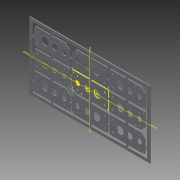
# Autodesk Inventor part: Granny Gearbox Input Plate Routing Template (9-up)
Saved by Autodesk Inventor 2015 (Build 190159000, 159)
## iProperties
Created: 2016-02-25
Part Number: Granny Gearbox Input Plate Routing Template (9-up)
Material: Generic
Document SubType Name: Modeling
Designer: sethbattis
Density: 1 g/cm^3
Appearance: Default
Author: sethbattis
Autodesk Inventor part; units mm, degrees
ref_plane "YZ Plane" through (0, 0, 0) normal (1, 0, 0) x (0, 1, 0)
ref_plane "XZ Plane" through (0, 0, 0) normal (0, 1, 0) x (-1, 0, 0)
ref_plane "XY Plane" through (0, 0, 0) normal (0, 0, 1) x (1, 0, 0)
derived "Granny Gearbox Input Plate.ipt"
feature "Solid1::Granny Gearbox Input Plate.ipt" [suppressed]
sketch "Shaft Alignment" plane through (0, 0, 0) normal (0, 0, 1) x (1, 0, 0)
  line L0 (-40.7035, -5.5985) -> (-0.0001, -11.1125) construction
  line L1 (-35.1409, -0.031) -> (-35.1353, -6.3528) construction
  line L2 (-11.1125, -0.0098) -> (-11.104, -9.6083) construction
  line L3 (0, 11.1125) -> (43.74, 13.9583) construction
  line L4 (-40.7035, -5.5985) -> (-46.2661, -5.5985) construction
  line L5 (-40.7035, -19.8733) -> (-46.2661, -19.8733) construction
  line L6 (-40.7035, 19.8015) -> (-46.2661, 19.8015) construction
  line L7 (-40.7035, 5.5267) -> (-46.2661, 5.5267) construction
  line L8 (-46.2661, 25.3641) -> (-46.2661, -25.4359) construction
  line L9 (-40.7035, 25.3641) -> (-40.7035, -25.4359) construction
  line L10 (-40.7035, -0.0359) -> (0, 0) construction
  line L11 (0, 0) -> (40.6908, 0) construction
  line L12 (11.1125, 0) -> (11.1125, 11.8355) construction
  line L13 (26.4033, 0) -> (26.4033, 12.8304) construction
  circle A0 centre (-40.7035, 25.3641) radius 5.5626
  circle A1 centre (-40.7035, -25.4359) radius 5.5626
  circle A2 centre (40.6908, 0) radius 14.2875
  circle A3 centre (0, 0) radius 11.1125
  circle A4 centre (-40.7035, -0.0359) radius 5.5626
  point P0 (-33.5787, -27.5177)
sketch "New Mounting Holes" plane through (0, 0, 0) normal (0, 0, 1) x (1, 0, 0)
  circle A0 centre (-40.7035, -0.0359) radius 31.75 construction
  circle A1 centre (40.6908, 0) radius 36.195 construction
  circle A2 centre (0, 0) radius 36.195 construction
  line L0 (-57.7242, 30.4609) -> (-55.8383, 30.4609) construction
  line L1 (-57.7242, 30.4609) -> (-57.7242, 28.575) construction
  circle A3 centre (-57.7242, 30.4609) radius 3.175
  circle A4 centre (-24.3812, -30.912) radius 3.175
  line L2 (-65.3633, -38.1) -> (-65.3633, 38.1) construction
  line L3 (87.0367, -38.1) -> (-65.3633, -38.1) construction
  line L4 (87.0367, 38.1) -> (87.0367, -38.1) construction
  line L5 (-65.3633, 38.1) -> (87.0367, 38.1) construction
  line L6 (-55.8383, 38.1) -> (-55.8383, -38.1) construction
  line L7 (-65.3633, 28.575) -> (87.0367, 28.575) construction
  line L8 (-65.3633, -28.575) -> (87.0367, -28.575) construction
  line L9 (77.5117, 38.1) -> (77.5117, -38.1) construction
  circle A5 centre (74.3367, 23.3553) radius 3.175
  circle A6 centre (74.3367, -23.3553) radius 3.175
sketch "Labels" plane through (0, 0, 0) normal (0, 0, 1) x (1, 0, 0)
  circle A0 centre (-40.7035, -0.0359) radius 5.5626
  circle A1 centre (-40.7035, 25.3641) radius 5.5626
  circle A2 centre (-40.7035, -25.4359) radius 5.5626
  circle A3 centre (0, 0) radius 11.1125
  circle A4 centre (40.6908, 0) radius 14.2875
  line L0 (-5.8677, 26.2224) -> (48.5566, 26.2224) construction
  line L1 (48.5566, 26.2224) -> (48.5566, 22.1963) construction
  line L2 (48.5566, 22.1963) -> (-5.8677, 22.1963) construction
  line L3 (-5.8677, 22.1963) -> (-5.8677, 26.2224) construction
sketch "Exterior" plane through (0, 0, 0) normal (0, 0, 1) x (1, 0, 0)
  line L0 (-65.3633, -17.4045) -> (-65.3633, 31.75)
  line L1 (-59.0133, 38.1) -> (80.6867, 38.1)
  line L2 (87.0367, 31.75) -> (87.0367, -31.75)
  line L3 (80.6867, -38.1) -> (-44.6678, -38.1)
  arc A0 (87.0367, 31.75) -> (80.6867, 38.1) centre (80.6867, 31.75) ccw
  arc A1 (80.6867, -38.1) -> (87.0367, -31.75) centre (80.6867, -31.75) ccw
  arc A2 (-59.0133, 38.1) -> (-65.3633, 31.75) centre (-59.0133, 31.75) ccw
  circle A3 centre (-40.7035, -0.0359) radius 31.75 construction
  line L4 (-63.5034, -21.8946) -> (-49.1579, -36.2401)
  line L5 (-65.3633, -38.1) -> (-65.3633, 38.1) construction
  line L6 (87.0367, -38.1) -> (-65.3633, -38.1) construction
  arc A4 (-49.1579, -36.2401) -> (-44.6678, -38.1) centre (-44.6678, -31.75) ccw
  arc A5 (-65.3633, -17.4045) -> (-63.5034, -21.8946) centre (-59.0133, -17.4045) ccw
  point P0 (87.0367, 38.1)
  point P1 (-65.3633, -20.0348)
  point P2 (-47.2981, -38.1)
sketch "Input Labels" plane through (0, 0, 0) normal (0, 0, 1) x (1, 0, 0)
  circle A0 centre (-40.7035, 25.3641) radius 2.667
  circle A1 centre (-40.7035, -0.0359) radius 9.525
  circle A2 centre (-40.7035, -25.4359) radius 2.667
  circle A3 centre (0, 0) radius 11.1125
  line L0 (-5.8677, 22.1963) -> (-5.8677, 26.2224) construction
  line L1 (-5.8677, 26.2224) -> (48.5566, 26.2224) construction
  line L2 (48.5566, 26.2224) -> (48.5566, 22.1963) construction
  line L3 (48.5566, 22.1963) -> (-5.8677, 22.1963) construction
  circle A4 centre (40.6908, 0) radius 14.2875
  line L4 (-5.8677, 26.2224) -> (45.7507, 26.2224) construction
  line L5 (45.7507, 26.2224) -> (45.7507, 22.1963) construction
  line L6 (45.7507, 22.1963) -> (-5.8677, 22.1963) construction
  line L7 (-5.8677, 22.1963) -> (-5.8677, 26.2224) construction
sketch "Sketch6" plane through (0, 0, 0) normal (0, 0, 1) x (1, 0, 0)
  line L0 (-63.5034, -21.8946) -> (-49.1579, -36.2401) projected
  line L1 (87.0367, -38.1) -> (-65.3633, -38.1) construction
  line L2 (87.0367, 38.1) -> (87.0367, -38.1) construction
  circle A0 centre (0, 0) radius 11.1125 projected
  circle A1 centre (40.6908, 0) radius 14.2875 projected
  circle A2 centre (-40.7035, 25.3641) radius 2.667 projected
  circle A3 centre (-40.7035, -0.0359) radius 9.525 projected
  circle A4 centre (-40.7035, -25.4359) radius 2.667 projected
  circle A5 centre (-24.3812, -30.912) radius 3.175 projected
  circle A6 centre (-57.7242, 30.4609) radius 3.175 projected
  circle A7 centre (74.3367, -23.3553) radius 3.175 projected
  line L3 (-58.0057, 37.3062) -> (5.249, 37.3062)
  line L4 (86.243, 30.9563) -> (86.243, 15.0813)
  line L5 (79.893, -37.3062) -> (19.5445, -37.3062)
  line L6 (-65.3633, 38.1) -> (87.0367, 38.1) construction
  line L7 (-65.3633, -38.1) -> (-65.3633, 38.1) construction
  line L8 (-62.4958, -21.7797) -> (-48.8291, -35.4464)
  line L9 (-64.3557, -17.2896) -> (-64.3557, 0.7938)
  circle A8 centre (-40.7035, -0.0359) radius 10.3187
  circle A9 centre (0, 0) radius 11.9062
  circle A10 centre (40.6908, 0) radius 15.0812
  circle A11 centre (0, 0) radius 36.195 construction
  arc A12 (86.243, 30.9563) -> (79.893, 37.3063) centre (79.893, 30.9563) ccw
  arc A13 (-58.0057, 37.3062) -> (-64.3557, 30.9562) centre (-58.0057, 30.9562) ccw
  arc A14 (-64.3557, -17.2896) -> (-62.4958, -21.7797) centre (-58.0057, -17.2896) ccw
  arc A15 (-48.8291, -35.4464) -> (-44.339, -37.3063) centre (-44.339, -30.9563) ccw
  arc A16 (79.893, -37.3062) -> (86.243, -30.9562) centre (79.893, -30.9562) ccw
  circle A17 centre (74.3367, 23.3553) radius 3.175 projected
  line L10 (9.2147, 41.1199) -> (9.2217, 41.3004)
  line L11 (9.2217, 41.3004) -> (15.5717, 41.3004)
  line L12 (15.5717, 41.3004) -> (15.5768, 41.4301)
  line L13 (9.2167, -41.4301) -> (9.2217, -41.3004)
  line L14 (9.2217, -41.3004) -> (15.5717, -41.3004)
  line L15 (15.5717, -41.3004) -> (15.5788, -41.1199)
  line L16 (90.2117, 4.7625) -> (90.2371, 4.7625)
  line L17 (90.2371, 4.7625) -> (90.2371, 11.1125)
  line L18 (90.2371, 11.1125) -> (90.2117, 11.1125)
  line L19 (-68.3244, 4.7625) -> (-68.5637, 4.7625)
  line L20 (-68.5637, 4.7625) -> (-68.5637, 11.1125)
  line L21 (-68.5637, 11.1125) -> (-68.3244, 11.1125)
  line L22 (19.5425, 37.3063) -> (79.893, 37.3063)
  line L23 (-64.3557, 15.0813) -> (-64.3557, 30.9562)
  line L24 (5.251, -37.3062) -> (-44.339, -37.3063)
  line L25 (86.243, 0.7938) -> (86.243, -30.9562)
  arc A18 (5.249, 37.3062) -> (9.2147, 41.1199) centre (5.249, 41.275) ccw
  arc A19 (15.5768, 41.4301) -> (19.5425, 37.3063) centre (19.5425, 41.275) ccw
  arc A20 (9.2167, -41.4301) -> (5.251, -37.3062) centre (5.251, -41.275) ccw
  arc A21 (19.5445, -37.3062) -> (15.5788, -41.1199) centre (19.5445, -41.275) ccw
  arc A22 (90.2117, 4.7625) -> (86.243, 0.7938) centre (90.2117, 0.7938) ccw
  arc A23 (86.243, 15.0813) -> (90.2117, 11.1125) centre (90.2117, 15.0813) ccw
  arc A24 (-68.3244, 11.1125) -> (-64.3557, 15.0813) centre (-68.3244, 15.0813) ccw
  arc A25 (-64.3557, 0.7938) -> (-68.3244, 4.7625) centre (-68.3244, 0.7938) ccw
  line L26 (9.2217, 41.3004) -> (9.2217, -41.3004) construction
  line L27 (-68.5637, 11.1125) -> (90.2371, 11.1125) construction
  point P0 (15.4156, 37.3062)
  dimension "d20" = 0.7937
  dimension "d23" = 0.7937
  dimension "d24" = 0.7937
  dimension "d25" = 19.05
  dimension "d26" = 20.6375
  dimension "d27" = 22.225
  dimension "d28" = 23.8125
  dimension "d29" = 28.575
  dimension "d30" = 30.1625
  dimension "d31" = 6.35
  dimension "d34" = 3.9942
  dimension "d35" = 3.9942
  dimension "d36" = 3.9942
  dimension "d38" = 0.7937
  dimension "d39" = 3.9688
  dimension "d40" = 6.35
  constraints: 46 end point, 34 tangent, 26 point on circle, 16 centre point, 13 parallel, 11 equal radius, 6 perpendicular, 5 horizontal, 3 coincident, 3 equal length, 3 point on line, 1 collinear, 1 vertical
  measures "d20" distance between parallel lines of L3 L6
  measures "d23" distance between parallel lines of L2 L4
  measures "d24" distance between parallel lines of L0 L8
  measures "d25" diameter of A3
  measures "d26" diameter of A8
  measures "d27" diameter of A0
  measures "d28" diameter of A9
  measures "d29" diameter of A1
  measures "d30" diameter of A10
  measures "d31" radius of A12
  measures "d34" distance between parallel lines of L3 L11
  measures "d35" distance between parallel lines of L5 L14
  measures "d36" distance between parallel lines of L4 L17
  measures "d38" distance between parallel lines of L24 L1
  measures "d39" radius of A18
  measures "d40" distance of L10.end L11.end
extrude "Extrusion2" add sketch "Sketch6" along normal blind 3.175 contours L3 A18 L10 L11 L12 A19 L22 A12 L4 A23 L18 L17 L16 A22 L25 A16 L5 A21 L15 L14 L13 A20 L24 A15 L8 A14 L9 A25 L19 L20 L21 A24 L23 A13
mirror "Mirror1" about plane through (90.2371, 4.7625, 0) normal (1, 0, 0) of "Extrusion2"
mirror "Mirror2" about plane through (-68.5637, 11.1125, 0) normal (-1, 0, 0) of "Extrusion2"
mirror "Mirror3" about plane through (15.5717, 41.3004, 0) normal (0, 1, 0) of "Extrusion2", "Mirror1", "Mirror2"
mirror "Mirror4" about plane through (-146.3491, -41.3004, 0) normal (0, -1, 0) of "Extrusion2", "Mirror2", "Mirror1"
sketch "Sketch7" plane through (0, 0, 0) normal (0, 0, 1) x (1, 0, 0)
  line L0 (-244.0586, -141.3256) -> (-244.0586, 141.3256)
  line L1 (-231.3586, -128.6256) -> (-231.3586, -97.6821)
  line L2 (-227.3645, 77.8383) -> (-227.3645, 71.4883) projected
  line L3 (-227.3645, -87.3633) -> (-227.3899, -87.3633)
  line L4 (-227.3645, -93.7133) -> (-227.3899, -93.7133)
  line L5 (-231.3586, -83.3946) -> (-231.3586, 0.7938)
  arc A0 (-231.3586, -83.3946) -> (-227.3899, -87.3633) centre (-227.3899, -83.3946) ccw
  arc A1 (-227.3899, -93.7133) -> (-231.3586, -97.6821) centre (-227.3899, -97.6821) ccw
  line L6 (-227.3645, 11.1125) -> (-227.3899, 11.1125)
  line L7 (-227.3645, 4.7625) -> (-227.3899, 4.7625)
  line L8 (-231.3586, 15.0813) -> (-231.3586, 67.5195)
  arc A2 (-231.3586, 15.0813) -> (-227.3899, 11.1125) centre (-227.3899, 15.0813) ccw
  arc A3 (-227.3899, 4.7625) -> (-231.3586, 0.7938) centre (-227.3899, 0.7938) ccw
  line L9 (-227.3645, 77.8383) -> (-227.3899, 77.8383)
  line L10 (-227.3645, 71.4883) -> (-227.3899, 71.4883)
  line L11 (-231.3586, 81.807) -> (-231.3586, 128.6256)
  arc A4 (-231.3586, 81.807) -> (-227.3899, 77.8383) centre (-227.3899, 81.807) ccw
  arc A5 (-227.3899, 71.4883) -> (-231.3586, 67.5195) centre (-227.3899, 67.5195) ccw
  line L12 (-227.3645, -87.3633) -> (-227.3645, -93.7133) projected
  line L13 (-227.3645, 4.7625) -> (-227.3645, 11.1125) projected
  line L14 (-227.3645, -87.3633) -> (-227.3645, -93.7133)
  line L15 (-227.3645, -93.7133) -> (-227.3391, -93.7133) projected
  line L16 (-227.3645, 11.1125) -> (-227.3645, 4.7625)
  line L17 (-227.3645, 11.1125) -> (-227.3645, 4.7625) projected
  line L18 (-227.3645, 77.8383) -> (-227.3645, 71.4883)
  line L19 (-244.0586, 141.3256) -> (-231.3586, 128.6256)
  line L20 (-231.3586, -128.6256) -> (-244.0586, -141.3256)
  point P0 (-146.3491, 123.9012)
  point P1 (-152.6991, 123.9012)
  point P2 (-152.6991, -123.9012)
  point P3 (-146.3491, -123.9012)
  point P4 (249.0379, 11.1125)
  point P5 (249.0379, 4.7625)
  point P6 (249.0379, 77.8383)
  dimension "d47" = 3.9942
  dimension "d59" = 3.9688
  dimension "d60" = 3.9688
  dimension "d61" = 3.9688
  constraints: 32 end point, 16 perpendicular, 15 tangent, 12 point on circle, 6 centre point, 3 equal radius, 1 collinear, 1 horizontal, 1 vertical
  measures "d47" distance between parallel lines of L2 L1
  measures "d59" radius of A0
  measures "d60" radius of A2
  measures "d61" radius of A4
extrude "Extrusion3" add sketch "Sketch7" along normal blind 3.175
ref_plane "Work Plane1" through (10.9436, -17.2896, 0) normal (-1, 0, 0) x (0, 0, 1)
mirror "Mirror5" about plane through (10.9436, -17.2896, 0) normal (-1, 0, 0) of "Extrusion3"
sketch "Sketch8" plane through (0, 0, 0) normal (0, 0, 1) x (1, 0, 0)
  line L0 (-146.3491, 123.9012) -> (-152.6991, 123.9012) projected
  line L1 (9.2217, 123.9012) -> (15.5717, 123.9012) projected
  line L2 (171.2525, 123.9012) -> (164.9025, 123.9012) projected
  line L3 (0, 197.8558) -> (0, -197.8558) projected
  line L4 (-244.0586, 141.3256) -> (265.9459, 141.3256)
  line L5 (265.9459, 141.3256) -> (265.9459, 128.6256)
  line L6 (265.9459, 128.6256) -> (-244.0586, 128.6256)
  line L7 (-244.0586, 128.6256) -> (-244.0586, 141.3256)
  line L8 (-152.6991, 123.9012) -> (-146.3491, 123.9012)
  line L9 (-146.3491, 123.9012) -> (-146.3491, 128.6256)
  line L10 (-146.3491, 128.6256) -> (-152.6991, 128.6256)
  line L11 (-152.6991, 128.6256) -> (-152.6991, 123.9012)
  line L12 (9.2217, 123.9012) -> (15.5717, 123.9012)
  line L13 (15.5717, 123.9012) -> (15.5717, 128.6256)
  line L14 (15.5717, 128.6256) -> (9.2217, 128.6256)
  line L15 (9.2217, 128.6256) -> (9.2217, 123.9012)
  line L16 (164.9025, 123.9012) -> (171.2525, 123.9012)
  line L17 (171.2525, 123.9012) -> (171.2525, 128.6256)
  line L18 (171.2525, 128.6256) -> (164.9025, 128.6256)
  line L19 (164.9025, 128.6256) -> (164.9025, 123.9012)
  line L20 (265.9459, 141.3256) -> (265.9459, -141.3256) projected
  point P0 (0, 0)
  constraints: 32 end point, 8 parallel, 4 horizontal, 4 perpendicular, 4 point on line, 2 collinear
extrude "Extrusion4" add sketch "Sketch8" along normal blind 3.175
ref_plane "Work Plane3" through (19.5425, 0, 0) normal (0, 1, 0) x (1, 0, 0)
mirror "Mirror6" about plane through (19.5425, 0, 0) normal (0, 1, 0) of "Extrusion4"
equation "\"d23\" = d20"
equation "\"d24\" = d20"
equation "\"d26\" = d25 + 2 * d20"
equation "\"d28\" = d27 + 2 * d20"
equation "\"d30\" = d29 + 2 * d20"
equation "\"d35\" = d34"
equation "\"d36\" = d34"
equation "\"d38\" = d20"
equation "\"d47\" = d34"
body "Solid1"
